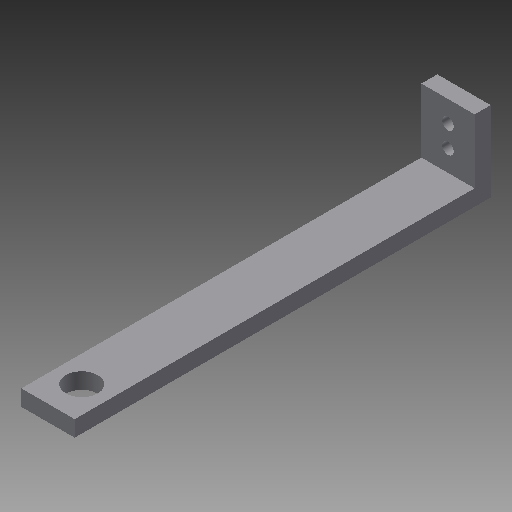
# Autodesk Inventor part: ALPHA_001158_Electrode8-mountbracket
Saved by Autodesk Inventor 2017 (Build 210142000, 142)
## iProperties
Created: 2015-11-18
Part Number: ALPHA_001158_Electrode8-mountbracket
Material: Generic
Document SubType Name: Modeling
Designer: massen
Density: 1 g/cm^3
Appearance: Default
Author: massen
Autodesk Inventor part; units mm, degrees
ref_plane "YZ Plane" through (0, 0, 0) normal (1, 0, 0) x (0, 1, 0)
ref_plane "XZ Plane" through (0, 0, 0) normal (0, 1, 0) x (-1, 0, 0)
ref_plane "XY Plane" through (0, 0, 0) normal (0, 0, 1) x (1, 0, 0)
sketch "Sketch1" plane through (0, 0, 0) normal (0, 1, 0) x (-1, 0, 0)
  line L0 (-4.2784, 62.5876) -> (5.7216, 62.5876)
  line L1 (5.7216, 62.5876) -> (5.7216, -15.4124)
  line L2 (5.7216, -15.4124) -> (-4.2784, -15.4124)
  line L3 (-4.2784, -15.4124) -> (-4.2784, 62.5876)
  line L4 (-4.2784, -15.4124) -> (5.7216, -15.4124)
  line L5 (5.7216, -15.4124) -> (5.7216, -12.4124)
  line L6 (5.7216, -12.4124) -> (-4.2784, -12.4124)
  line L7 (-4.2784, -12.4124) -> (-4.2784, -15.4124)
  circle A0 centre (0.7216, 56.2526) radius 3
  point P0 (0, 0)
  dimension "d0" = 10
  dimension "d1" = 78
  dimension "d2" = 6.335
  dimension "d3" = 3
  dimension "d16" = 6
  constraints: 16 end point, 4 parallel, 2 horizontal, 2 perpendicular, 1 centre point, 1 point on line
  measures "d0" distance between parallel lines of L1 L3
  measures "d1" distance between parallel lines of L0 L2
  measures "d2" distance from line of L0 A0.centre
  measures "d3" distance between parallel lines of L2 L6
  measures "d16" diameter of A0
extrude "Extrusion1" add sketch "Sketch1" along normal blind 3 contours L0 L1 L6 L3
extrude "Extrusion2" add sketch "Sketch1" along normal blind 15 contours L6 L1 L2 L3
sketch "Sketch2" plane through (-5.7216, 3, -12.4124) normal (0, 0, 1) x (1, 0, 0)
  line L0 (0, 0) -> (0, 12) projected
  line L1 (0, 0) -> (10, 0) projected
  line L2 (5, 4) -> (5, 8) construction
  point P0 (5.7216, -3)
  point P1 (5, 0)
  point P2 (0, 6)
  point P3 (5, 6)
  dimension "d8" = 4
  constraints: 3 midpoint, 2 end point, 2 vertical alignment, 1 horizontal alignment, 1 perpendicular
  measures "d8" distance of L2.start L2.end
hole "Hole1" at (-0.7216, 11, -12.4124) at (-0.7216, 7, -12.4124) direction (0, 0, -1) diameter 2.2 end through all
body "Solid1"
